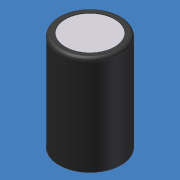
# Autodesk Inventor part: Capacitor
Saved by Autodesk Inventor 2011 SP1 (Build 150282100, 282)
## iProperties
Shininess: 64.0
Length Units: 11272
Angle Units: 11279
Time Units: 11290
Mass Units: 11286
Length Display Precision: 3
Angle Display Precision: 2
Compacted: True
Part Number: Capacitor
Document SubType Name: Modeling
Created: 2007-01-15
Designer: uidk0133
Density: 1 g/cm^3
Density: 0.0
Volumn: 0.0
Area: 0.0
PropertySet Name: Model Information
Control State: 0
Master: False
Checked Out: False
Author: uidk0133
Autodesk Inventor part; units mm, degrees
ref_plane "YZ Plane" through (0, 0, 0) normal (1, 0, 0) x (0, 1, 0)
ref_plane "XZ Plane" through (0, 0, 0) normal (0, 1, 0) x (-1, 0, 0)
ref_plane "XY Plane" through (0, 0, 0) normal (0, 0, 1) x (1, 0, 0)
sketch "Sketch1" plane through (0, 0, 0) normal (0, 0, 1) x (1, 0, 0)
  circle A0 centre (0, 0) radius 6.35
  dimension "d0" = 12.7
  constraints: 1 centre point
  measures "d0" diameter of A0
extrude "Extrusion1" add sketch "Sketch1" along normal mid plane 20.32
fillet "Fillet1" radius 0.635 1 edges at (-6.35, 0, 10.16)
sketch "Sketch2" plane through (0, 0, 10.16) normal (0, 0, 1) x (1, 0, 0)
  circle A0 centre (0, 0) radius 5.715 projected
  circle A1 centre (0, 0) radius 5.0354
  constraints: 1 centre point, 1 coincident, 1 concentric
extrude "Extrusion2" cut sketch "Sketch2" against normal blind 0.127 contours A1
body "Solid1"
